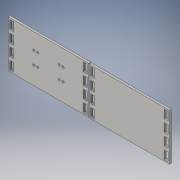
# Autodesk Inventor part: RTS New Frame
Saved by Autodesk Inventor 2016 (Build 200138000, 138)
## iProperties
Created: 2017-10-04
Part Number: RTS New Frame
Material: Generic
Document SubType Name: Modeling
Designer: student
Density: 1 g/cm^3
Appearance: Default
Author: student
Autodesk Inventor part; units mm, degrees
ref_plane "YZ Plane" through (0, 0, 0) normal (1, 0, 0) x (0, 1, 0)
ref_plane "XZ Plane" through (0, 0, 0) normal (0, 1, 0) x (-1, 0, 0)
ref_plane "XY Plane" through (0, 0, 0) normal (0, 0, 1) x (1, 0, 0)
sketch "Sketch1" plane through (0, 0, 0) normal (0, 0, 1) x (1, 0, 0)
  circle A0 centre (17.8867, 8.4338) radius 1.2446
  circle A1 centre (17.8867, -7.0602) radius 1.2446
  circle A2 centre (13.1877, -7.0602) radius 1.2446
  circle A3 centre (13.1877, 8.4338) radius 1.2446
  line L0 (42.1828, 26.035) -> (42.1828, 15.875)
  line L1 (42.1828, 15.875) -> (46.8818, 15.875)
  line L2 (46.8818, 15.875) -> (46.8818, 26.035)
  line L3 (42.1828, 26.035) -> (46.8818, 26.035)
  line L4 (48.6598, 27.813) -> (48.6598, -28.575)
  line L5 (42.1828, 1.651) -> (46.8818, 1.651)
  line L6 (42.1828, 11.811) -> (42.1828, 1.651)
  line L7 (46.8818, 1.651) -> (46.8818, 11.811)
  line L8 (42.1828, 11.811) -> (46.8818, 11.811)
  line L9 (42.1828, -12.573) -> (46.8818, -12.573)
  line L10 (42.1828, -2.413) -> (42.1828, -12.573)
  line L11 (46.8818, -12.573) -> (46.8818, -2.413)
  line L12 (42.1828, -2.413) -> (46.8818, -2.413)
  line L13 (42.1828, -26.797) -> (46.8818, -26.797)
  line L14 (42.1828, -16.637) -> (42.1828, -26.797)
  line L15 (46.8818, -26.797) -> (46.8818, -16.637)
  line L16 (42.1828, -16.637) -> (46.8818, -16.637)
  line L17 (-41.8018, 26.035) -> (-41.8018, 15.875)
  line L18 (-41.8018, 15.875) -> (-46.5008, 15.875)
  line L19 (-46.5008, 15.875) -> (-46.5008, 26.035)
  line L20 (-41.8018, 26.035) -> (-46.5008, 26.035)
  line L21 (-48.2788, 27.813) -> (-48.2788, -28.575)
  line L22 (-41.8018, 1.651) -> (-46.5008, 1.651)
  line L23 (-41.8018, 11.811) -> (-41.8018, 1.651)
  line L24 (-46.5008, 1.651) -> (-46.5008, 11.811)
  line L25 (-41.8018, 11.811) -> (-46.5008, 11.811)
  line L26 (-41.8018, -12.573) -> (-46.5008, -12.573)
  line L27 (-41.8018, -2.413) -> (-41.8018, -12.573)
  line L28 (-46.5008, -12.573) -> (-46.5008, -2.413)
  line L29 (-41.8018, -2.413) -> (-46.5008, -2.413)
  line L30 (-41.8018, -26.797) -> (-46.5008, -26.797)
  line L31 (-41.8018, -16.637) -> (-41.8018, -26.797)
  line L32 (-46.5008, -26.797) -> (-46.5008, -16.637)
  line L33 (-41.8018, -16.637) -> (-46.5008, -16.637)
  line L34 (-48.2788, 27.813) -> (48.6598, 27.813)
  line L35 (-48.2788, -28.575) -> (48.6598, -28.575)
  line L36 (139.7308, 25.654) -> (139.7308, 15.494)
  line L37 (139.7308, 15.494) -> (144.4298, 15.494)
  line L38 (144.4298, 15.494) -> (144.4298, 25.654)
  line L39 (139.7308, 25.654) -> (144.4298, 25.654)
  line L40 (146.2078, 27.432) -> (146.2078, -28.956)
  line L41 (139.7308, 1.27) -> (144.4298, 1.27)
  line L42 (139.7308, 11.43) -> (139.7308, 1.27)
  line L43 (144.4298, 1.27) -> (144.4298, 11.43)
  line L44 (139.7308, 11.43) -> (144.4298, 11.43)
  line L45 (139.7308, -12.954) -> (144.4298, -12.954)
  line L46 (139.7308, -2.794) -> (139.7308, -12.954)
  line L47 (144.4298, -12.954) -> (144.4298, -2.794)
  line L48 (139.7308, -2.794) -> (144.4298, -2.794)
  line L49 (139.7308, -27.178) -> (144.4298, -27.178)
  line L50 (139.7308, -17.018) -> (139.7308, -27.178)
  line L51 (144.4298, -27.178) -> (144.4298, -17.018)
  line L52 (139.7308, -17.018) -> (144.4298, -17.018)
  line L53 (55.7462, 15.494) -> (51.0472, 15.494)
  line L54 (55.7462, 25.654) -> (55.7462, 15.494)
  line L55 (51.0472, 15.494) -> (51.0472, 25.654)
  line L56 (55.7462, 25.654) -> (51.0472, 25.654)
  line L57 (55.7462, 11.43) -> (55.7462, 1.27)
  line L58 (51.0472, 1.27) -> (51.0472, 11.43)
  line L59 (55.7462, 11.43) -> (51.0472, 11.43)
  line L60 (55.7462, 1.27) -> (51.0472, 1.27)
  line L61 (55.7462, -2.794) -> (55.7462, -12.954)
  line L62 (51.0472, -12.954) -> (51.0472, -2.794)
  line L63 (55.7462, -2.794) -> (51.0472, -2.794)
  line L64 (55.7462, -12.954) -> (51.0472, -12.954)
  line L65 (55.7462, -17.018) -> (51.0472, -17.018)
  line L66 (55.7462, -17.018) -> (55.7462, -27.178)
  line L67 (51.0472, -27.178) -> (51.0472, -17.018)
  line L68 (55.7462, -27.178) -> (51.0472, -27.178)
  line L69 (49.2692, 27.432) -> (49.2692, -28.956)
  line L70 (49.2692, 27.432) -> (146.2078, 27.432)
  line L71 (49.2692, -28.956) -> (146.2078, -28.956)
  circle A4 centre (-17.5057, -7.0602) radius 1.2446
  circle A5 centre (-17.5057, 8.4338) radius 1.2446
  circle A6 centre (-12.8067, -7.0602) radius 1.2446
  circle A7 centre (-12.8067, 8.4338) radius 1.2446
  point P0 (0, 0)
  point P1 (0, 0)
  point P2 (0, 0)
  point P3 (0, 0)
  point P4 (0, 0)
  point P5 (0, 0)
  point P6 (0, 0)
  point P7 (0, 0)
  point P8 (0, 0)
  point P9 (0, 0)
  point P10 (0, 0)
  point P11 (0, 0)
  point P12 (0, 0)
  point P13 (0, 0)
  point P14 (0, 0)
  point P15 (0, 0)
  point P16 (97.548, -0.381)
  point P17 (97.548, -0.381)
  point P18 (97.548, -0.381)
  point P19 (97.548, -0.381)
  point P20 (97.548, -0.381)
  point P21 (97.548, -0.381)
  point P22 (97.548, -0.381)
  point P23 (97.548, -0.381)
  point P24 (97.548, -0.381)
  point P25 (97.548, -0.381)
  point P26 (97.548, -0.381)
  point P27 (97.548, -0.381)
  point P28 (97.548, -0.381)
  point P29 (97.548, -0.381)
  point P30 (97.548, -0.381)
  dimension "d2" = 2.4892
  dimension "d3" = 2.4892
  dimension "d5" = 15.494
  dimension "d7" = 2.4892
  dimension "d8" = 2.4892
  dimension "d9" = 15.494
  dimension "d10" = 4.699
  dimension "d19" = 4.699
  dimension "d23" = 4.699
  dimension "d24" = 10.16
  dimension "d145" = 14.224
  dimension "d190" = 10.16
  dimension "d192" = 1.778
  dimension "d212" = 1.778
  dimension "d215" = 1.778
  dimension "d216" = 4.064
  dimension "d217" = 4.064
  dimension "d218" = 4.064
  dimension "d219" = 10.16
  dimension "d220" = 10.16
  dimension "d221" = 10.16
  dimension "d222" = 4.064
  dimension "d223" = 1.778
  dimension "d268" = 4.699
  dimension "d269" = 10.16
  dimension "d270" = 14.224
  dimension "d271" = 10.16
  dimension "d272" = 1.778
  dimension "d273" = 1.778
  dimension "d274" = 1.778
  dimension "d275" = 4.064
  dimension "d276" = 4.064
  dimension "d277" = 4.064
  dimension "d278" = 10.16
  dimension "d279" = 10.16
  dimension "d280" = 10.16
  dimension "d281" = 4.064
  dimension "d282" = 1.778
  constraints: 144 end point, 8 centre point, 6 horizontal, 2 collinear, 2 parallel, 2 perpendicular, 2 vertical, 46 other
  measures "d2" diameter of A1
  measures "d3" diameter of A0
  measures "d5" distance of A1.centre A0.centre
  measures "d7" diameter of A2
  measures "d8" diameter of A3
  measures "d9" distance of A2.centre A3.centre
  measures "d10" distance of A0.centre A3.centre
  measures "d19" distance of A1.centre A2.centre
  measures "d23" distance of L2.end L0.start
  measures "d24" distance of L0.start L0.end
  measures "d145" distance of L0.end L5.start
  measures "d190" distance of L17.start L18.start
  measures "d192" distance between parallel lines of L21 L19
  measures "d212" distance between parallel lines of L34 L20
  measures "d215" distance between parallel lines of L35 L30
  measures "d216" distance between parallel lines of L33 L26
  measures "d217" distance between parallel lines of L29 L22
  measures "d218" distance between parallel lines of L25 L18
  measures "d219" distance of L23.start L23.end
  measures "d220" distance of L27.start L27.end
  measures "d221" distance of L33.start L31.end
  measures "d222" distance between parallel lines of L1 L8
  measures "d223" distance between parallel lines of L35 L13
  measures "d268" distance of L39.end L36.start
  measures "d269" distance of L36.start L36.end
  measures "d270" distance of L36.end L42.end
  measures "d271" distance of L56.start L53.start
  measures "d272" distance between parallel lines of L69 L55
  measures "d273" distance between parallel lines of L70 L56
  measures "d274" distance between parallel lines of L71 L68
  measures "d275" distance between parallel lines of L65 L64
  measures "d276" distance between parallel lines of L63 L60
  measures "d277" distance between parallel lines of L59 L53
  measures "d278" distance of L57.start L57.end
  measures "d279" distance of L61.start L61.end
  measures "d280" distance of L66.start L66.end
  measures "d281" distance between parallel lines of L37 L44
  measures "d282" distance between parallel lines of L71 L49
extrude "Extrusion13" add sketch "Sketch1" along normal blind 2.54
body "Solid13"
